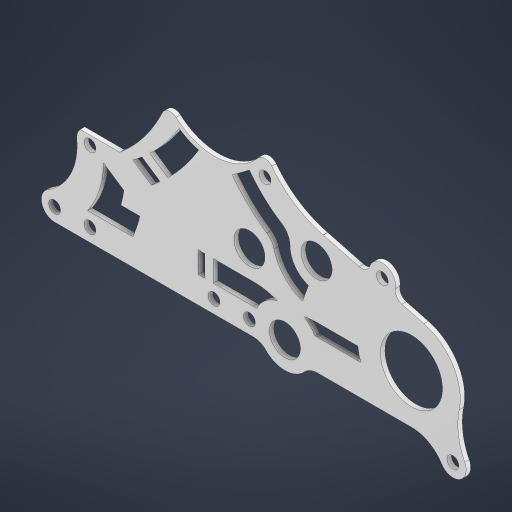
# Autodesk Inventor part: reservoir_mount_inner
Saved by Autodesk Inventor 2024 (Build 280153000, 153)
## iProperties
Created: 2023-11-18
Part Number: reservoir_mount_inner
Material: Acetal Resin, White
Document SubType Name: Sheet Metal
Designer: avere
Density: 1.425 g/cm^3
Appearance: Smooth - White
Flat Pattern Width: 6.54287 cm
Flat Pattern Length: 15.2289 cm
Flat Pattern Area: 99.6407 cm^2
Sheet Metal Rule: Default_mm
Sheet Metal Width: 2.576 in
Sheet Metal Length: 5.996 in
Sheet Metal Area: 15.444 in^2
Author: avere
Autodesk Inventor part; units mm, degrees
ref_plane "YZ Plane" through (0, 0, 0) normal (1, 0, 0) x (0, 1, 0)
ref_plane "XZ Plane" through (0, 0, 0) normal (0, 1, 0) x (-1, 0, 0)
ref_plane "XY Plane" through (0, 0, 0) normal (0, 0, 1) x (1, 0, 0)
sketch "main" plane through (0, 0, 0) normal (0, 0, 1) x (1, 0, 0)
  circle A0 centre (-14.2783, -9.7185) radius 2.1844
  ellipse E0 centre (34.925, 23.8125) end of major axis (34.925, 33.3375) minor radius 9.5235
  point P0 (-4.2471, 2.7063)
sketch "Sketch1" plane through (0, 0, 0) normal (0, 0, 1) x (1, 0, 0)
  arc A0 (-3.5163, 3.212) -> (-4.7431, -0.4299) centre (0, 0) ccw
  circle A1 centre (0, -25.4) radius 2.0955
  circle A2 centre (-12.7, -25.4) radius 2.0955
  arc A3 (-15.2019, -21.3476) -> (-12.7, -30.1625) centre (-12.7, -25.4) ccw
  line L0 (-12.7, -30.1625) -> (-11.7807, -30.1625)
  arc A4 (-15.2019, -21.3476) -> (-4.7431, -0.4299) centre (-26.8773, -2.4363) ccw
  line L1 (31.75, -25.4) -> (57.15, -25.4) construction
  line L2 (31.75, -25.4) -> (36.5125, -25.4) construction
  circle A5 centre (44.45, -25.4) radius 2.0955
  circle A6 centre (57.15, -25.4) radius 2.0955
  circle A7 centre (69.85, -25.4) radius 5.5499
  arc A8 (63.0478, -32.0675) -> (76.8244, -31.8872) centre (69.85, -25.4) ccw
  circle A9 centre (57.15, -3.403) radius 5.5499
  line L3 (-11.7807, -30.1625) -> (58.513, -30.1625)
  line L4 (81.474, -29.8619) -> (115.2189, -29.8619)
  line L5 (-11.7807, -30.1625) -> (61.6011, -30.1625) construction
  line L6 (78.2653, -29.8619) -> (115.2189, -29.8619) construction
  circle A10 centre (81.2023, 4.7609) radius 5.5499
  arc A11 (83.6265, 13.9723) -> (83.523, 13.9989) centre (81.2023, 4.7609) ccw
  arc A12 (65.1561, 26.0829) -> (83.523, 13.9989) centre (91.6512, 46.3534) ccw
  arc A13 (81.474, -29.8619) -> (76.8244, -31.8872) centre (81.474, -36.2119) ccw
  arc A14 (63.0478, -32.0675) -> (58.513, -30.1625) centre (58.513, -36.5125) ccw
  circle A15 centre (115.2189, -12.3994) radius 11.0998
  arc A16 (132.3184, -15.9417) -> (119.6634, 4.488) centre (115.2189, -12.3994) ccw
  circle A17 centre (104.775, 11.1125) radius 2.0955
  arc A18 (109.4545, 10.2271) -> (100.2659, 12.6454) centre (104.775, 11.1125) ccw
  line L7 (119.6634, 4.488) -> (111.766, 6.5664)
  line L8 (96.4518, 10.5969) -> (83.6265, 13.9723)
  arc A19 (96.4518, 10.5969) -> (100.2659, 12.6454) centre (97.2599, 13.6673) ccw
  arc A20 (109.4545, 10.2271) -> (111.766, 6.5664) centre (112.5741, 9.6369) ccw
  circle A21 centre (130.0641, -33.3375) radius 2.0955
  arc A22 (126.0228, -35.8574) -> (134.3205, -31.2011) centre (130.0641, -33.3375) ccw
  arc A23 (132.3184, -15.9417) -> (134.3205, -31.2011) centre (155.2553, -20.6933) ccw
  arc A24 (126.0228, -35.8574) -> (115.2189, -29.8619) centre (115.2189, -42.5941) ccw
  arc A25 (122.2659, -20.9753) -> (122.2726, -21.4129) centre (155.2553, -20.6933) ccw
  arc A26 (59.7857, -20.6886) -> (58.513, -20.6375) centre (58.513, -36.5125) ccw
  arc A27 (-0.8623, -20.6375) -> (4.8666, -3.0564) centre (-26.8773, -2.4363) ccw
  arc A28 (67.0849, -14.637) -> (58.513, -13.0175) centre (58.513, -36.5125) ccw
  arc A29 (11.0441, -13.0175) -> (12.1111, -7.9042) centre (-26.8773, -2.4363) ccw
  line L9 (4.8666, -3.0564) -> (12.1111, -7.9042)
  line L10 (18.5803, 5.7275) -> (25.1468, 1.3334)
  line L11 (21.4396, 8.2742) -> (27.9161, 3.9403)
  arc A30 (15.3458, -20.6375) -> (17.8676, -13.0175) centre (-26.8773, -2.4363) ccw
  line L12 (17.8676, -13.0175) -> (11.0441, -13.0175)
  line L13 (15.3458, -20.6375) -> (-0.8623, -20.6375)
  line L14 (38.7856, -20.6375) -> (38.7856, -13.0175)
  line L15 (41.1925, -20.6375) -> (41.1925, -13.0175)
  line L16 (44.2415, -13.0175) -> (44.2415, -20.6375)
  line L17 (58.513, -13.0175) -> (44.2415, -13.0175)
  line L18 (41.1925, -13.0175) -> (38.7856, -13.0175)
  line L19 (58.513, -20.6375) -> (44.2415, -20.6375)
  line L20 (41.1925, -20.6375) -> (38.7856, -20.6375)
  arc A31 (41.2533, 43.0681) -> (41.1925, 43.0108) centre (44.4887, 39.5733) ccw
  line L21 (15.3458, 3.189) -> (22.0356, -1.2876)
  arc A32 (15.3458, 3.189) -> (18.5803, 5.7275) centre (-22.4149, 54.6332) ccw
  arc A33 (21.4396, 8.2742) -> (31.9538, 21.2204) centre (-22.4149, 54.6332) ccw
  arc A34 (22.0356, -1.2876) -> (25.1468, 1.3334) centre (-22.4149, 54.6332) ccw
  line L22 (51.0183, 16.3583) -> (57.1143, 20.9307)
  arc A35 (40.5702, 20.9307) -> (41.1925, 20.8107) centre (44.4887, 39.5733) ccw
  arc A36 (27.9161, 3.9403) -> (38.9427, 18.0514) centre (-22.4149, 54.6332) ccw
  arc A37 (83.6265, 13.9723) -> (83.523, 13.9989) centre (81.2023, 4.7609) ccw
  arc A38 (71.6773, 4.7523) -> (78.3204, -4.3176) centre (81.2023, 4.7609) ccw
  arc A39 (65.9685, 0.8308) -> (76.1756, -10.147) centre (81.2023, 4.7609) ccw
  arc A40 (51.0183, 16.3583) -> (63.375, 4.506) centre (91.6512, 46.3534) ccw
  arc A41 (57.1143, 20.9307) -> (68.7224, 10.1128) centre (91.6512, 46.3534) ccw
  arc A42 (112.1958, -29.8619) -> (117.1762, -30.0133) centre (115.2189, -12.3994) ccw
  arc A43 (67.0849, -14.637) -> (59.7857, -20.6886) centre (69.85, -25.4) ccw
  arc A44 (59.8098, -30.1625) -> (59.882, -30.3118) centre (69.85, -25.4) ccw
  arc A45 (79.9432, -30.0492) -> (80.0274, -29.8619) centre (69.85, -25.4) ccw
  arc A46 (81.474, -14.2875) -> (76.801, -14.7913) centre (81.474, -36.2119) ccw
  arc A47 (80.6713, -18.7848) -> (76.801, -14.7913) centre (69.85, -25.4) ccw
  arc A48 (81.474, -18.7664) -> (80.6713, -18.7848) centre (81.474, -36.2119) ccw
  line L23 (81.474, -18.7664) -> (97.0069, -18.7664)
  arc A49 (96.0187, -14.2875) -> (97.0069, -18.7664) centre (115.2189, -12.3994) ccw
  line L24 (96.0187, -14.2875) -> (81.474, -14.2875)
  circle A50 centre (62.7575, 21.436) radius 2.0955
  line L25 (78.3204, -4.3176) -> (76.1756, -10.147)
  arc A51 (71.6773, 4.7523) -> (68.7224, 10.1128) centre (65.3273, 4.7466) ccw
  arc A52 (65.9685, 0.8308) -> (63.375, 4.506) centre (59.8198, -0.7554) ccw
  arc A53 (10.6679, 3.212) -> (25.8705, 23.0519) centre (-26.8733, 47.7228) ccw
  arc A54 (30.8454, 24.0889) -> (60.215, 26.2096) centre (44.4887, 39.5733) ccw
  arc A55 (31.9538, 21.2204) -> (38.9427, 18.0514) centre (44.4887, 39.5733) ccw
  arc A56 (30.8454, 24.0889) -> (25.8705, 23.0519) centre (28.7464, 21.7067) ccw
  arc A57 (65.1561, 26.0829) -> (60.215, 26.2096) centre (62.6345, 24.1537) ccw
  circle A58 centre (0, 0) radius 2.0955
  line L26 (-3.5163, 3.212) -> (10.6679, 3.212)
  point P0 (-1.8077, 4.4061)
  point P1 (63.0492, 4.0753)
  point P2 (107.9569, 7.5689)
  point P3 (100.2609, 9.5944)
  point P4 (9.126, 4.4208)
  point P5 (41.1925, 20.8107)
  dimension "d7" = 22.225
  dimension "d25" = 4.191
  dimension "d26" = 4.191
  dimension "d30" = 11.0998
  dimension "d31" = 11.0998
  dimension "d38" = 6.35
  dimension "d43" = 4.191
  dimension "d44" = 9.525
  dimension "d47" = 9.525
  dimension "d54" = 4.191
  dimension "d55" = 6.35
  dimension "d56" = 12.7
  dimension "d58" = 41.275
  dimension "d60" = 3.175
  constraints: 102 point on circle, 58 centre point, 54 end point, 28 tangent, 14 horizontal, 11 coincident, 9 point on line, 6 perpendicular, 4 equal radius, 3 parallel, 1 concentric, 1 midpoint, 11 other
  measures "d7" radius of A4
  measures "d25" diameter of A5
  measures "d26" diameter of A6
  measures "d30" diameter of A7
  measures "d31" diameter of A9
  measures "d38" radius of A13
  measures "d43" diameter of A17
  measures "d44" diameter of A18
  measures "d47" diameter of A22
  measures "d54" diameter of A50
  measures "d55" radius of A51
  measures "d56" distance of L26.start point (9.126, 4.421)
  measures "d58" diameter of A54
  measures "d60" radius of A56
extrude "Extrusion1" add sketch "Sketch1" along normal blind 1.5875 contours L26 A53 A56 A54 A57 A12 A11 L8 A19 A18 A20 L7 A16 A23 A22 A24 L4 A13 A8 A14 L3 L0 A3 A4 A0
body "Solid1"
